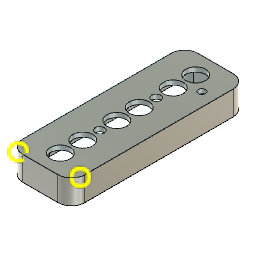
Nixie Tube Clock (Autodesk Fusion 360 design; units mm, degrees)
part number: 2025-11-05-12-53-28-767
Autodesk Fusion 360 part; units mm, degrees
sketch "Sketch1" plane through (0, 0, 0) normal (0, 0, 1) x (1, 0, 0)
  line L0 (10, 0) -> (59, 0)
  line L1 (69, 10) -> (69, 170)
  line L2 (59, 180) -> (10, 180)
  line L3 (0, 170) -> (0, 10)
  arc A0 (10, 180) -> (0, 170) centre (10, 170) ccw
  arc A1 (69, 170) -> (59, 180) centre (59, 170) ccw
  arc A2 (59, 0) -> (69, 10) centre (59, 10) ccw
  arc A3 (0, 10) -> (10, 0) centre (10, 10) ccw
  point P0 (69, 0)
  point P1 (0, 180)
  dimension "d1" = 69
  dimension "d2" = 180
  dimension "d3" = 10
  dimension "d4" = 10
  dimension "d5" = 10
  constraint horizontal L0
  constraint vertical L1
  constraint horizontal L2
  constraint vertical L3
  constraint coincident P1 L2
  constraint coincident P1 L3
  constraint tangent L2 A0
  constraint tangent L3 A0
  constraint tangent L1 A1
  constraint tangent L2 A1
  constraint coincident P0 L1
  constraint coincident P0 L0
  constraint tangent L1 A2
  constraint tangent L0 A2
  constraint equal A1 A2
  constraint coincident origin L0
  constraint coincident origin L3
  constraint tangent L0 A3
  constraint tangent L3 A3
  measures "d1" distance of origin P0
  measures "d2" distance of origin P1
  measures "d3" radius of A0
  measures "d4" radius of A1
  measures "d5" radius of A3
sketch "Sketch2" plane through (0, 0, 27) normal (0, 0, 1) x (-1, 0, 0)
  line L0 (-10, 0) -> (-59, 0)
  arc A0 (-59, 0) -> (-69, -10) centre (-59, -10) ccw
sketch "Sketch3" plane through (0, 0, 0) normal (0, 0, 1) x (1, 0, 0)
  line L0 (15, 0) -> (54, 0)
  line L1 (69, 15) -> (69, 180)
  line L2 (54, 195) -> (15, 195)
  line L3 (0, 180) -> (0, 15)
  circle A0 centre (34.5, 110) radius 11
  circle A1 centre (34.5, 85) radius 11
  circle A2 centre (34.5, 128.9) radius 5
  circle A3 centre (34.5, 66.1) radius 5
  circle A4 centre (34.5, 47.2) radius 11
  circle A5 centre (34.5947, 147.7998) radius 11
  circle A6 centre (34.5, 22.2) radius 11
  circle A7 centre (34.4989, 172.7996) radius 11
  arc A8 (15, 195) -> (0, 180) centre (15, 180) ccw
  arc A9 (69, 180) -> (54, 195) centre (54, 180) ccw
  arc A10 (54, 0) -> (69, 15) centre (54, 15) ccw
  arc A11 (0, 15) -> (15, 0) centre (15, 15) ccw
  circle A12 centre (54, 160.2997) radius 4
  point P0 (69, 0)
  dimension "d76" = 22
  dimension "d77" = 22
  dimension "d78" = 18.9
  dimension "d79" = 18.9
  dimension "d80" = 10
  dimension "d81" = 10
  dimension "d82" = 18.9
  dimension "d83" = 18.9
  dimension "d84" = 22
  dimension "d85" = 22
  dimension "d86" = 25
  dimension "d87" = 25
  dimension "d88" = 22
  dimension "d89" = 22
  dimension "d90" = 15
  dimension "d91" = 15
  dimension "d92" = 15
  dimension "d93" = 15
  dimension "d130" = 8
  constraint horizontal L0
  constraint vertical L1
  constraint horizontal L2
  constraint vertical L3
  constraint tangent L2 A8
  constraint tangent L3 A8
  constraint tangent L1 A9
  constraint tangent L2 A9
  constraint coincident P0 L0
  constraint coincident P0 L1
  constraint tangent L0 A10
  constraint tangent L1 A10
  constraint tangent L3 A11
  constraint tangent L0 A11
  measures "d76" diameter of A0
  measures "d77" diameter of A1
  measures "d78" distance of A0.centre A2.centre
  measures "d79" distance of A1.centre A3.centre
  measures "d80" diameter of A2
  measures "d81" diameter of A3
  measures "d82" distance of A2.centre A5.centre
  measures "d83" distance of A3.centre A4.centre
  measures "d84" diameter of A4
  measures "d85" diameter of A5
  measures "d86" distance of A5.centre A7.centre
  measures "d87" distance of A4.centre A6.centre
  measures "d88" diameter of A6
  measures "d89" diameter of A7
  measures "d90" radius of A8
  measures "d91" radius of A9
  measures "d92" radius of A10
  measures "d93" radius of A11
  measures "d130" diameter of A12
sketch "Sketch4" plane through (0, 0, 27) normal (0, 0, 1) x (-1, 0, 0)
sketch "Sketch5" plane through (0, 0, 0) normal (0, 0, 1) x (1, 0, 0)
extrude "Extrude2" add sketch "Sketch3" along normal blind 27
sketch "Sketch6" plane through (0, 0, 0) normal (0, 0, -1) x (1, 0, 0)
  circle A0 centre (54, -160.2997) radius 4
  circle A1 centre (34.4989, -172.7996) radius 11
  circle A2 centre (34.5, -110) radius 11
  circle A3 centre (34.5947, -147.7998) radius 11
  circle A4 centre (34.5, -85) radius 11
  circle A5 centre (34.5, -66.1) radius 5
  circle A6 centre (34.5, -47.2) radius 11
  circle A7 centre (34.5, -22.2) radius 11
  circle A8 centre (34.5, -128.9) radius 5
  arc A9 (15, 0) -> (0, -15) centre (15, -15) ccw
  line L0 (0, -15) -> (0, -180)
  arc A10 (0, -180) -> (15, -195) centre (15, -180) ccw
  line L1 (15, -195) -> (54, -195)
  arc A11 (54, -195) -> (69, -180) centre (54, -180) ccw
  line L2 (69, -180) -> (69, -15)
  arc A12 (69, -15) -> (54, 0) centre (54, -15) ccw
  line L3 (54, 0) -> (15, 0)
  line L4 (34.5, -85) -> (0, -85)
  line L5 (15, -5) -> (54, -5)
  line L6 (64, -15) -> (64, -180)
  line L7 (54, -190) -> (15, -190)
  line L8 (5, -180) -> (5, -15)
  arc A13 (15, -5) -> (5, -15) centre (15, -15) ccw
  arc A14 (64, -15) -> (54, -5) centre (54, -15) ccw
  arc A15 (5, -180) -> (15, -190) centre (15, -180) ccw
  arc A16 (54, -190) -> (64, -180) centre (54, -180) ccw
  dimension "d162" = 10
  dimension "d163" = 10
  dimension "d164" = 10
  dimension "d165" = 10
  constraint coincident A4.centre L4.start
  constraint coincident L0 L4.end
  constraint perpendicular L0 L4
  constraint horizontal L5
  constraint vertical L6
  constraint horizontal L7
  constraint vertical L8
  constraint tangent L5 A13
  constraint tangent L8 A13
  constraint tangent L5 A14
  constraint tangent L6 A14
  constraint tangent L7 A15
  constraint tangent L8 A15
  constraint tangent L7 A16
  constraint tangent L6 A16
  measures "d162" radius of A13
  measures "d163" radius of A14
  measures "d165" radius of A16
extrude "Extrude3" cut sketch "Sketch6" against normal blind 22 contours L5 L6 L7 L8 A13 A14 A15 A16
sketch "Sketch7" plane through (0, 0, 27) normal (0, 0, 1) x (-1, 0, 0)
  circle A0 centre (-54, -160.2997) radius 4
  circle A1 centre (-34.4989, -172.7996) radius 11
  circle A2 centre (-34.5, -110) radius 11
  circle A3 centre (-34.5947, -147.7998) radius 11
  circle A4 centre (-34.5, -85) radius 11
  circle A5 centre (-34.5, -66.1) radius 5
  circle A6 centre (-34.5, -47.2) radius 11
  circle A7 centre (-34.5, -22.2) radius 11
  circle A8 centre (-34.5, -128.9) radius 5
  arc A9 (0, -15) -> (-15, 0) centre (-15, -15) ccw
  line L0 (-15, 0) -> (-54, 0)
  arc A10 (-54, 0) -> (-69, -15) centre (-54, -15) ccw
  line L1 (-69, -15) -> (-69, -180)
  arc A11 (-69, -180) -> (-54, -195) centre (-54, -180) ccw
  line L2 (-54, -195) -> (-15, -195)
  arc A12 (-15, -195) -> (0, -180) centre (-15, -180) ccw
  line L3 (0, -180) -> (0, -15)
sketch "Sketch8" plane through (0, 0, 0) normal (0, 0, -1) x (1, 0, 0)
  line L0 (54, -190) -> (15, -190)
  arc A0 (5, -180) -> (15, -190) centre (15, -180) ccw
  line L1 (5, -180) -> (5, -15)
  arc A1 (15, -5) -> (5, -15) centre (15, -15) ccw
  line L2 (15, -5) -> (54, -5)
  arc A2 (64, -15) -> (54, -5) centre (54, -15) ccw
  line L3 (64, -15) -> (64, -180)
  arc A3 (54, -190) -> (64, -180) centre (54, -180) ccw
  arc A4 (15, 0) -> (0, -15) centre (15, -15) ccw
  line L4 (0, -15) -> (0, -180)
  arc A5 (0, -180) -> (15, -195) centre (15, -180) ccw
  line L5 (15, -195) -> (54, -195)
  arc A6 (54, -195) -> (69, -180) centre (54, -180) ccw
  line L6 (69, -180) -> (69, -15)
  arc A7 (69, -15) -> (54, 0) centre (54, -15) ccw
  line L7 (54, 0) -> (15, 0)
  line L8 (0, -34.7) -> (0, -29.7)
  line L9 (0, -34.7) -> (0, -39.7)
  line L10 (0, -39.7) -> (0, -29.7)
  line L11 (0, -29.7) -> (5, -29.7)
  line L12 (0, -39.7) -> (5, -39.7)
  line L13 (5, -29.7) -> (5, -39.7)
  constraint parallel L4 L9
  constraint parallel L8 L10
  constraint coincident L1 L11.end
  constraint perpendicular L1 L11
  constraint coincident L1 L12.end
  constraint perpendicular L1 L12
extrude "Extrude4" cut sketch "Sketch8" against normal blind 5 contours L1 L4 L8 L9 L10 L11 L12 L13
sketch "Sketch9" plane through (0, 0, 0) normal (-1, 0, 0) x (0, -1, 0)
  line L0 (-39.7, 0) -> (-39.7, 5)
  line L1 (-39.7, 5) -> (-29.7, 5)
  line L2 (-29.7, 5) -> (-29.7, 0)
  line L3 (-29.7, 0) -> (-15, 0)
  line L4 (-15, 0) -> (-15, 27)
  line L5 (-15, 27) -> (-180, 27)
  line L6 (-180, 27) -> (-180, 0)
  line L7 (-180, 0) -> (-39.7, 0)
  line L8 (-29.7, 0) -> (-29.7, 3)
  line L9 (-31.7, 5) -> (-37.7, 5)
  line L10 (-39.7, 3) -> (-39.7, 0)
  arc A0 (-29.7, 3) -> (-31.7, 5) centre (-31.7, 3) ccw
  arc A1 (-37.7, 5) -> (-39.7, 3) centre (-37.7, 3) ccw
  dimension "d176" = 2
  dimension "d177" = 2
  constraint coincident L2.end L3.start
  constraint coincident L0.start L7.end
  constraint tangent L8 A0
  constraint tangent L9 A0
  constraint tangent L10 A1
  constraint tangent L9 A1
  measures "d176" radius of A0
  measures "d177" radius of A1
extrude "Extrude5" add sketch "Sketch9" against normal blind 5 contours L0 L1 A1 | L1 L2 A0
sketch "Sketch10" plane through (0, 0, 0) normal (-1, 0, 0) x (0, -1, 0)
  line L0 (-39.7, 0) -> (-39.7, 3)
  arc A0 (-37.7, 5) -> (-39.7, 3) centre (-37.7, 3) ccw
  line L1 (-37.7, 5) -> (-31.7, 5)
  arc A1 (-29.7, 3) -> (-31.7, 5) centre (-31.7, 3) ccw
  line L2 (-29.7, 3) -> (-29.7, 0)
  line L3 (-29.7, 0) -> (-15, 0)
  line L4 (-15, 0) -> (-15, 27)
  line L5 (-15, 27) -> (-180, 27)
  line L6 (-180, 27) -> (-180, 0)
  line L7 (-180, 0) -> (-39.7, 0)
